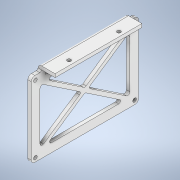
# Autodesk Inventor part: batteryBracket
Saved by Autodesk Inventor 2022 (Build 260153000, 153)
## iProperties
Created: 2022-04-12
Part Number: batteryBracket
Material: PC/ABS Plastic
Document SubType Name: Modeling
Designer: Dahway
Mass: 22.0736 g
Surface Area: 159.209 cm^2
Volume: 22.0736 cm^3
Density: 0.357273 g/cm^3
Appearance: Smooth - White
Author: Dahway
Autodesk Inventor part; units mm, degrees
ref_plane "YZ Plane" through (0, 0, 0) normal (1, 0, 0) x (0, 1, 0)
ref_plane "XZ Plane" through (0, 0, 0) normal (0, 1, 0) x (-1, 0, 0)
ref_plane "XY Plane" through (0, 0, 0) normal (0, 0, 1) x (1, 0, 0)
sketch "Sketch1" plane through (0, 0, 0) normal (0, 1, 0) x (-1, 0, 0)
  line L0 (0, 0) -> (14.8, 0)
  line L1 (14.8, 0) -> (14.8, 75.4)
  line L2 (14.8, 75.4) -> (0, 75.4)
  line L3 (0, 75.4) -> (0, 0)
  dimension "d0" = 14.8
  dimension "d1" = 75.4
  constraints: 8 end point, 2 parallel, 1 horizontal, 1 perpendicular
  measures "d0" distance of L2.end L1.end
  measures "d1" distance of L1.end L0.end
extrude "Extrusion1" add sketch "Sketch1" along normal blind 40.7
sketch "Sketch2" plane through (0, 0, 0) normal (0, -1, 0) x (1, 0, 0)
  line L0 (0, 75.4) -> (0, 0) projected
  line L1 (-14.8, 75.4) -> (0, 75.4) projected
  line L2 (0, 0) -> (-11.8, 0)
  line L3 (-11.8, 0) -> (-11.8, 75.4)
  line L4 (-11.8, 75.4) -> (0, 75.4)
  line L5 (0, 75.4) -> (0, 0)
  dimension "d4" = 11.8
  constraints: 8 end point, 2 parallel, 1 horizontal, 1 perpendicular, 1 point on line
  measures "d4" distance of L3.end L4.end
extrude "Extrusion2" cut sketch "Sketch2" against normal blind 37.7
ref_plane "Work Plane1" through (0, 40.7, 37.7) normal (0, 0, -1) x (-1, 0, 0)
sketch "Sketch4" plane through (0, 37.7, 0) normal (0, -1, 0) x (1, 0, 0)
  circle A0 centre (-4, 3.7) radius 1.5
  circle A1 centre (-4, 6.5) radius 1.5
  line L0 (-5.5, 3.7) -> (-5.5, 6.5)
  line L1 (-2.5, 3.7) -> (-2.5, 6.5)
  line L2 (0, 0) -> (-11.8, 0) projected
  line L3 (0, 75.4) -> (0, 0) projected
  dimension "d17" = 3
  dimension "d18" = 3
  dimension "d19" = 3.7
  dimension "d20" = 4
  dimension "d21" = 2.8
  constraints: 4 end point, 4 point on circle, 2 centre point, 2 tangent, 1 parallel, 1 vertical
  measures "d17" diameter of A0
  measures "d18" diameter of A1
  measures "d19" distance from line of L2 A0.centre
  measures "d20" distance from line of L3 A0.centre
  measures "d21" distance of A1.centre A0.centre
extrude "Extrusion4" add sketch "Sketch4" along normal blind 3
fillet "Fillet1" radius 1 4 edges at (-4, 34.7, 2.2) (-2.5, 34.7, 5.1) (-4, 34.7, 8) (-5.5, 34.7, 5.1)
mirror "Mirror2" about plane through (0, 40.7, 37.7) normal (0, 0, -1) of "Extrusion4", "Fillet1"
sketch "Sketch22" plane through (0, 40.7, 0) normal (0, 1, 0) x (1, 0, 0)
  line L0 (-14.8, -75.4) -> (0, -75.4) projected
  line L1 (-7.8, -72.1) -> (-7.8, -75.4) projected
  line L2 (0, 0) -> (-14.8, 0) projected
  point P0 (-4, -59.3)
  point P1 (-3.9, -16.1)
  point P2 (-7.8, 0)
  dimension "d126" = 16.1
  dimension "d127" = 3.8
  dimension "d128" = 16.1
  measures "d126" distance from line of L0 point (-4, -59.3)
  measures "d127" distance from line of L1 point (-4, -59.3)
  measures "d128" distance from line of L2 point (-3.9, -16.1)
hole "Hole2" at (-4, 40.7, 59.3) at (-3.9, 40.7, 16.1) direction (0, -1, 0) diameter 3.15 depth 3 tip angle 118
sketch "Sketch24" plane through (-14.8, 0, 0) normal (-1, 0, 0) x (0, 0, 1)
  line L0 (84.25, 36.285) -> (-8.85, 36.285)
  line L1 (-8.85, 36.285) -> (-8.85, -28.915)
  line L2 (-8.85, -28.915) -> (84.25, -28.915)
  line L3 (84.25, -28.915) -> (84.25, 36.285)
  point P0 (0, 0)
  dimension "d170" = 93.1
  dimension "d171" = 65.2
  dimension "d172" = 36.285
  dimension "d173" = 8.85
  constraints: 8 end point, 2 parallel, 1 horizontal, 1 perpendicular
  measures "d170" distance of L2.end L1.end
  measures "d171" distance of L1.end L0.end
  measures "d172" distance from line of point (0, 0) L0
  measures "d173" distance from line of point (0, 0) L1
extrude "Extrusion19" add sketch "Sketch24" against normal up to surface (3 mm away)
sketch "Sketch25" plane through (-14.8, 40.7, 0) normal (-1, 0, 0) x (0, 0, 1)
  line L0 (-8.85, -4.415) -> (-8.85, -69.615) projected
  line L1 (84.25, -69.615) -> (84.25, -4.415) projected
  line L2 (-8.85, -69.615) -> (84.25, -69.615) projected
  point P0 (0, -40.7)
  point P1 (-5.35, -7.915)
  point P2 (-5.3498, -66.115)
  point P3 (80.75, -66.315)
  point P4 (80.7498, -8.115)
  dimension "d176" = 86.1
  dimension "d177" = 3.5
  dimension "d178" = 58.2
  dimension "d179" = 3.5
  dimension "d180" = 58.2
  dimension "d181" = 86.1
  dimension "d182" = 3.5
  dimension "d183" = 3.3
  measures "d176" distance of point (80.75, -8.115) point (-5.35, -7.915)
  measures "d177" distance from line of L0 point (-5.35, -7.915)
  measures "d178" distance of point (-5.35, -66.115) point (-5.35, -7.915)
  measures "d179" horizontal distance of L0.start point (-5.35, -7.915)
  measures "d180" distance of point (80.75, -66.315) point (80.75, -8.115)
  measures "d181" distance of point (-5.35, -66.115) point (80.75, -66.315)
  measures "d182" distance from line of L1 point (80.75, -66.315)
  measures "d183" distance from line of L2 point (80.75, -66.315)
hole "Hole3" at (-14.8, 32.585, 80.7498) at (-14.8, -25.415, -5.3498) at (-14.8, -25.615, 80.75) at (-14.8, 32.785, -5.35) direction (1, 0, 0) diameter 3.15 end through all
fillet "Fillet14" radius 3.15 5 edges at (-13.3, 36.285, -8.85) (-14.8, 40.7, 37.7) (-13.3, 36.285, 84.25) (-13.3, -28.915, 84.25) (-13.3, -28.915, -8.85)
sketch "Sketch26" plane through (-14.8, -25.765, -8.85) normal (-1, 0, 0) x (0, 0, 1)
  line L0 (7.5, 54.35) -> (85.6, 54.35)
  line L1 (85.6, 54.35) -> (85.6, 4.35)
  line L2 (85.6, 4.35) -> (7.5, 4.35)
  line L3 (7.5, 4.35) -> (7.5, 54.35)
  line L4 (7.5, 54.35) -> (85.6, 4.35) construction
  line L5 (85.6, 54.35) -> (7.5, 4.35) construction
  line L6 (0, 58.9) -> (0, 0) projected
  line L7 (3.15, -3.15) -> (89.95, -3.15) projected
  point P0 (8.85, 25.765)
  point P1 (46.55, 29.35)
  dimension "d192" = 78.1
  dimension "d193" = 50
  dimension "d194" = 7.5
  dimension "d195" = 7.5
  constraints: 12 end point, 2 midpoint, 2 parallel, 1 horizontal, 1 perpendicular
  measures "d192" distance of L1.end L2.end
  measures "d193" distance of L0.end L1.end
  measures "d194" distance between parallel lines of L6 L3
  measures "d195" distance between parallel lines of L7 L2
extrude "Extrusion20" cut sketch "Sketch26" against normal up to surface (3 mm away)
sketch "Sketch27" plane through (0, 37.7, 0) normal (0, -1, 0) x (1, 0, 0)
  line L0 (-11.8, 0) -> (-11.8, 75.4) projected
  line L1 (-11.8, 68.9) -> (-7.7, 68.9)
  line L2 (-7.7, 68.9) -> (-7.7, 6.5)
  line L3 (-7.7, 6.5) -> (-11.8, 6.5)
  line L4 (-11.8, 6.5) -> (-11.8, 68.9)
  line L5 (-14.1737, 0) -> (0, 0) projected
  point P0 (-11.8, -0.5209)
  point P1 (-11.8, 75.9209)
  dimension "d198" = 4.1
  dimension "d199" = 62.4
  dimension "d200" = 6.5
  constraints: 8 end point, 2 parallel, 1 horizontal, 1 perpendicular, 1 point on line
  measures "d198" distance of L2.end L3.end
  measures "d199" distance of L1.end L2.end
  measures "d200" distance between parallel lines of L5 L3
extrude "Extrusion21" add sketch "Sketch27" along normal blind 5
fillet "Fillet15" radius 3.15 4 edges at (-11.8, 35.2, 6.5) (-7.7, 35.2, 6.5) (-11.8, 35.2, 68.9) (-7.7, 35.2, 68.9)
fillet "Fillet16" radius 3.15 4 edges at (-13.3, 28.585, -1.35) (-13.3, 28.585, 76.75) (-13.3, -21.415, 76.75) (-13.3, -21.415, -1.35)
sketch "Sketch28" plane through (-14.8, -25.765, 84.25) normal (-1, 0, 0) x (0, 0, 1)
  circle A0 centre (-89.6, 58.55) radius 1.575 projected
  line L0 (-88.7159, 59.8535) -> (-2.6159, 1.4535)
  circle A1 centre (-3.5, 0.15) radius 1.575 projected
  line L1 (-90.4841, 57.2465) -> (-4.3841, -1.1535)
  circle A2 centre (-89.6, 58.55) radius 1.575 projected
  line L2 (-84.25, 63.315) -> (-8.85, 63.315) projected
  line L3 (-10.65, 4.35) -> (-82.45, 4.35) projected
  circle A3 centre (-89.5998, 0.35) radius 1.575 projected
  line L4 (-90.4797, 1.6563) -> (-4.3802, 59.6563)
  circle A4 centre (-3.5002, 58.35) radius 1.575 projected
  line L5 (-88.7198, -0.9563) -> (-2.6203, 57.0437)
  point P0 (-84.25, 25.765)
  point P1 (-43.7376, 29.3455)
  point P2 (-46.547, 31.2511)
  point P3 (-49.3624, 29.3545)
  point P4 (-46.553, 27.4489)
  constraints: 8 end point, 8 point on circle, 8 tangent
extrude "Extrusion22" add sketch "Sketch28" against normal up to surface (3 mm away) contours A0 L0 L4 L1 | L4 A4 L5 L0 | L0 L5 L1 L4 | L1 L5 A3 L4 | L0 A1 L1 L5
fillet "Fillet17" radius 1.415 2 edges at (-13.3, 36.285, 75.4) (-13.3, 36.285, 0)
fillet "Fillet18" radius 2 6 edges at (-13.3, 27.5903, -0.4972) (-13.3, -20.3123, -0.594) (-13.3, -20.4203, 75.8972) (-13.3, 27.4823, 75.994) (-13.3, 5.4861, 37.703) (-13.3, 1.6839, 37.697)
fillet "Fillet19" radius 1.5 6 edges at (-13.3, -21.415, 3.4072) (-13.3, -21.415, 71.7521) (-13.3, 28.585, 71.9928) (-13.3, 28.585, 3.6479) (-13.3, 3.5895, 34.8876) (-13.3, 3.5805, 40.5124)
body "Solid1"
